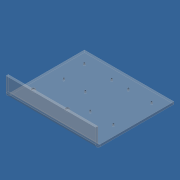
# Autodesk Inventor part: P1704_009
Saved by Autodesk Inventor 2015 SP2 (Build 190223200, 223)
## iProperties
Created: 2018-05-15
Part Number: P1704_009
Project: Nom Projet
Material: Plastique PMMA
Description: Nom pièce
Document SubType Name: Tôlerie
Designer: Alexandre.PICOTTE
Authority: brut Ø
Sheet Metal Rule: Par défaut
Appearance: Transparent - Clair
Material number: ---
Author: Alexandre.PICOTTE
Autodesk Inventor part; units mm, degrees
ref_plane "Plan YZ" through (0, 0, 0) normal (1, 0, 0) x (0, 1, 0)
ref_plane "Plan XZ" through (0, 0, 0) normal (0, 1, 0) x (-1, 0, 0)
ref_plane "Plan XY" through (0, 0, 0) normal (0, 0, 1) x (1, 0, 0)
sketch "Esquisse1" plane through (0, 0, 0) normal (0, 0, 1) x (1, 0, 0)
  line L0 (-78, 70) -> (78, 70)
  line L1 (80, 68) -> (80, -68)
  line L2 (78, -70) -> (-78, -70)
  line L3 (-80, -68) -> (-80, 68)
  line L4 (-112, 0) -> (112, 0) construction
  line L5 (0, -98) -> (0, 98) construction
  line L6 (-80, 68) -> (-80, 70)
  line L7 (-80, 70) -> (-78, 70)
  line L8 (80, 68) -> (80, 70)
  line L9 (78, 70) -> (80, 70)
  line L10 (-78, -70) -> (-80, -70)
  line L11 (-80, -70) -> (-80, -68)
  line L12 (78, -70) -> (80, -70)
  line L13 (80, -70) -> (80, -68)
  point P0 (0, 0)
  dimension "d0" = 160
  dimension "d1" = 140
  constraints: 24 end point, 8 point on line, 5 perpendicular, 2 collinear, 2 horizontal, 2 parallel, 1 vertical, 2 other
  measures "d0" distance of L6.end L8.end
  measures "d1" distance of L10.end L6.end
extrude "Extrusion1" add sketch "Esquisse1" along normal blind 4
sketch "Esquisse5" plane through (0, 0, 4) normal (0, 0, 1) x (1, 0, 0)
  line L0 (18.6, 50) -> (60, 50) construction
  line L1 (60, 50) -> (60, -18.2) construction
  line L2 (60, -18.2) -> (18.6, -18.2) construction
  line L3 (18.6, -18.2) -> (18.6, 50) construction
  line L4 (80, -70.465) -> (80, 70)
  line L5 (80, 70) -> (-80, 70)
  line L6 (80, 70) -> (-80, 70) projected
  line L7 (80, -70) -> (80, 70) projected
  point P0 (0, 0)
  point P1 (0, 0)
  point P2 (78, 70)
  point P3 (-78, 70)
  point P4 (80, -68)
  point P5 (80, 68)
  dimension "d12" = 41.4
  dimension "d13" = 68.2
  dimension "d14" = 20
  dimension "d15" = 20
  constraints: 12 end point, 4 coincident, 2 collinear, 2 parallel, 1 horizontal, 1 perpendicular
  measures "d12" distance of L0.start L0.end
  measures "d13" distance of L2.end L0.start
  measures "d14" distance between parallel lines of L4 L1
  measures "d15" distance between parallel lines of L5 L0
hole "Perçage1" at (18.6, 50, 4) at (60, 50, 4) at (18.6, -18.2, 4) at (60, -18.2, 4) direction (0, 0, -1) diameter 2.459 end through all thread size "M3x0.5" class "6H" standard "ISO M"
sketch "Esquisse6" plane through (0, 0, 4) normal (0, 0, 1) x (1, 0, 0)
  line L0 (-60, 50) -> (-11.3, 50) construction
  line L1 (-11.3, 50) -> (-11.3, 8.1) construction
  line L2 (-11.3, 8.1) -> (-60, 8.1) construction
  line L3 (-60, 8.1) -> (-60, 50) construction
  line L4 (-35.65, 66.5768) -> (-35.65, 16.8329)
  line L5 (-80, 70) -> (-80, -63.3699)
  line L6 (-80, 70) -> (-80, -70) construction
  line L7 (80, 70) -> (-80, 70) projected
  circle A0 centre (18.6, 50) radius 1.2295 construction
  point P0 (0, 0)
  point P1 (0, 0)
  point P2 (-54.9, 8.1)
  point P3 (-16.4, 8.1)
  point P4 (-80, 68)
  point P5 (-80, -68)
  point P6 (78, 70)
  point P7 (-78, 70)
  dimension "d23" = 41.9
  dimension "d24" = 38.5
  dimension "d25" = 48.7
  dimension "d26" = 48.7
  dimension "d27" = 20
  constraints: 13 end point, 3 coincident, 3 point on line, 2 parallel, 1 collinear, 1 horizontal, 1 perpendicular, 1 symmetric about line, 1 vertical, 2 other
  measures "d23" distance of L2.end L0.start
  measures "d24" distance of point (-16.4, 8.1) point (-54.9, 8.1)
  measures "d25" diameter of L1 L4
  measures "d26" distance of L0.start L0.end
  measures "d27" distance between parallel lines of L5 L3
hole "Perçage2" at (-54.9, 8.1, 4) at (-16.4, 8.1, 4) at (-60, 50, 4) at (-11.3, 50, 4) direction (0, 0, -1) diameter 2.459 end through all thread size "M3x0.5" class "6H" standard "ISO M"
sketch "Esquisse7" plane through (0, 0, 4) normal (0, 0, 1) x (1, 0, 0)
  line L0 (-66.05, -35) -> (-5.25, -35) construction
  line L1 (78.7638, -70) -> (-80, -70)
  line L2 (-35.65, 25.8994) -> (-35.65, -17.0856) construction
  line L3 (-97.8207, -35) -> (11.6326, -35)
  line L4 (-80, 70) -> (-80, -70)
  line L5 (-80, 70) -> (-80, -70) projected
  line L6 (80, 70) -> (-80, 70) projected
  circle A0 centre (-16.4, 8.1) radius 1.2295 construction
  point P0 (0, 0)
  point P1 (0, 0)
  point P2 (-80, 68)
  point P3 (-80, -68)
  point P4 (78, 70)
  point P5 (-78, 70)
  dimension "d35" = 60.8
  dimension "d37" = 70
  dimension "d40" = 140
  dimension "d41" = 38.5
  constraints: 11 end point, 2 coincident, 2 horizontal, 1 collinear, 1 point on line, 1 symmetric about line, 1 vertical
  measures "d35" distance of L0.start L0.end
  measures "d37" diameter of L1 L3
  measures "d40" distance of L4.start L1.end
  measures "d41" diameter of A0.centre L2
hole "Perçage3" at (-66.05, -35, 4) at (-5.25, -35, 4) direction (0, 0, -1) diameter 3.4 end through all
sketch "Esquisse10" plane through (80, -66, 0) normal (0, -1, 0) x (1, 0, 0)
  line L0 (-160, 0) -> (0, 0)
  line L1 (0, 0) -> (0, 34)
  line L2 (0, 34) -> (-160, 34)
  line L3 (-160, 34) -> (-160, 0)
  constraints: 6 end point, 1 horizontal, 1 perpendicular, 1 vertical
edge flange "Bord tombé2" height 34 angle 90 thickness 4 bend radius 4 thickness toward (0, -1, 0) relief tear relief width 4 relief depth 2 edges at (0, -70, 4) wall of the first edge with corners at (-80, -66, 0) (80, -66, 0) (80, -66, 34) (-80, -66, 34)
bend "Pli3"
corner "Coin2"
sketch "Esquisse11" plane through (0, 0, 0) normal (0, 0, -1) x (-1, 0, 0)
  circle A0 centre (66.05, -35) radius 1.7 projected
  circle A1 centre (66.05, -35) radius 3.25
  circle A2 centre (5.25, -35) radius 1.7 projected
  circle A3 centre (5.25, -35) radius 3.25
  point P0 (0, 0)
  dimension "d75" = 6.5
  constraints: 2 centre point, 2 coincident, 1 equal radius
  measures "d75" diameter of A1
extrude "Extrusion2" cut sketch "Esquisse11" against normal blind 2.8
equation "\"d26\" = d25"
equation "\"d37\" = 0.5 * d39"
equation "\"d41\" = d24"
equation "\"d65\" = LargeurGrugeage"
equation "\"d66\" = ProfondeurGrugeage"
equation "\"d67\" = RestesMinimum"
equation "\"d68\" = RayonPli"
equation "\"d71\" = RayonPli"
equation "\"d72\" = TailleGrugeage"
equation "\"d73\" = TailleJeu"
equation "\"d74\" = TailleRayonJacobi"
equation "\"RayonPli\" = Epaisseur"
equation "\"LargeurGrugeage\" = Epaisseur"
equation "\"ProfondeurGrugeage\" = 0.5 * Epaisseur"
equation "\"TailleGrugeage\" = 4 * Epaisseur"
equation "\"RestesMinimum\" = 2 * Epaisseur"
equation "\"Rayondetransition\" = RayonPli"
equation "\"TailleRayonJacobi\" = Epaisseur"
equation "\"TailleJeu\" = Epaisseur"
equation "\"d39\" = 140"
equation "\"Epaisseur\" = 4"
